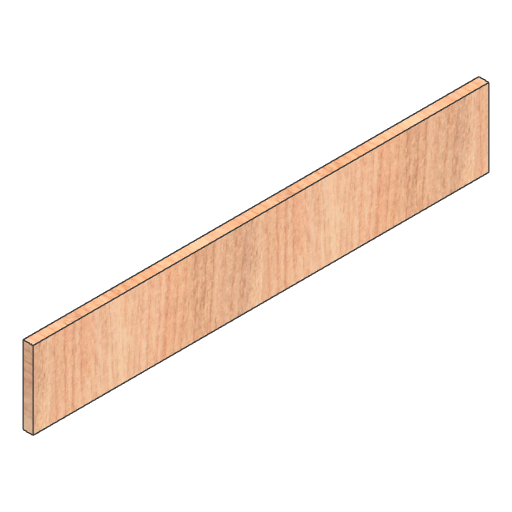
# Autodesk Inventor part: CUT PART N-01
Saved by Autodesk Inventor 2023.2 (Build 272271000, 271)
## iProperties
Created: 2022-11-08
Part Number: CUT PART N-01
Material: Wood (Birch)
Document SubType Name: Modeling
Designer: GUT
Density: 0.55 g/cm^3
Appearance: Birch - Natural Polished
Mass: 334.521 g
Surface Area: 1166.82 cm^2
Volume: 608.22 cm^3
d1: 93,000 mm
Author: GUT
Autodesk Inventor part; units mm, degrees
ref_plane "YZ Plane" through (0, 0, 0) normal (1, 0, 0) x (0, 1, 0)
ref_plane "XZ Plane" through (0, 0, 0) normal (0, 1, 0) x (-1, 0, 0)
ref_plane "XY Plane" through (0, 0, 0) normal (0, 0, 1) x (1, 0, 0)
sketch "Sketch1" plane through (0, 0, 0) normal (1, 0, 0) x (0, 1, 0)
  line L0 (455.1523, 757.311) -> (548.1523, 757.311)
  line L1 (548.1523, 757.311) -> (548.1523, 212.311)
  line L2 (548.1523, 212.311) -> (455.1523, 212.311)
  line L3 (455.1523, 212.311) -> (455.1523, 757.311)
  point P0 (0, 0)
  dimension "b" = 545
  dimension "d1" = 93
  constraints: 8 end point, 2 parallel, 1 horizontal, 1 perpendicular
  measures "b" distance of L0.end L1.end
  measures "d1" distance of L0.start L0.end
extrude "Extrusion1" add sketch "Sketch1" along normal blind 12
body "Solid1"
